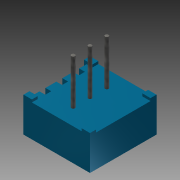
# Autodesk Inventor part: BasePotenciometro
Saved by Autodesk Inventor 2013 (Build 170138000, 138)
## iProperties
Created: 2013-06-26
Part Number: BasePotenciometro
Material: Genérico
Document SubType Name: Modeling
Designer: usuario
Density: 1 g/cm^3
Author: usuario
Autodesk Inventor part; units mm, degrees
ref_plane "YZ Plane" through (0, 0, 0) normal (1, 0, 0) x (0, 1, 0)
ref_plane "XZ Plane" through (0, 0, 0) normal (0, 1, 0) x (-1, 0, 0)
ref_plane "XY Plane" through (0, 0, 0) normal (0, 0, 1) x (1, 0, 0)
sketch "Boceto1" plane through (0, 0, 0) normal (0, 0, 1) x (1, 0, 0)
  line L0 (-4.78, 4.78) -> (4.78, 4.78)
  line L1 (4.78, 4.78) -> (4.78, -4.78)
  line L2 (4.78, -4.78) -> (-4.78, -4.78)
  line L3 (-4.78, -4.78) -> (-4.78, 4.78)
  line L4 (-4.78, 4.78) -> (4.78, -4.78) construction
  line L5 (4.78, 4.78) -> (-4.78, -4.78) construction
  point P0 (0, 0)
  dimension "d0" = 9.56
  dimension "d1" = 9.56
  constraints: 12 end point, 2 midpoint, 2 parallel, 1 horizontal, 1 perpendicular
  measures "d0" distance of L1.end L2.end
  measures "d1" distance of L0.end L1.end
extrude "Extrusión1" add sketch "Boceto1" along normal mid plane 4.6
sketch "Boceto2" plane through (0, 0, 2.3) normal (0, 0, 1) x (1, 0, 0)
  line L0 (-4.78, 4.78) -> (-3.58, 4.78)
  line L1 (-3.58, 4.78) -> (-3.58, 3.92)
  line L2 (-3.58, 3.92) -> (-4.78, 3.92)
  line L3 (-4.78, 3.92) -> (-4.78, 4.78)
  point P0 (0, 0)
  dimension "d4" = 1.2
  dimension "d5" = 0.86
  constraints: 8 end point, 2 parallel, 1 horizontal, 1 perpendicular
  measures "d4" distance of L1.end L2.end
  measures "d5" distance of L0.end L1.end
extrude "Extrusión2" add sketch "Boceto2" along normal blind 0.37
mirror "Simetría1" about plane through (0, 0, 0) normal (0, 1, 0) of "Extrusión2"
mirror "Simetría2" about plane through (0, 0, 0) normal (1, 0, 0) of "Extrusión2", "Simetría1"
sketch "Boceto5" plane through (0, 0, 2.3) normal (0, 0, 1) x (1, 0, 0)
  line L0 (-3.58, 3.92) -> (-4.78, 3.92) projected
  line L1 (-4.78, -3.92) -> (-4.41, -3.92)
  line L2 (-4.41, -3.92) -> (-4.41, 3.92)
  line L3 (-4.41, 3.92) -> (-4.78, 3.92)
  line L4 (-4.78, 3.92) -> (-4.78, -3.92)
  point P0 (0, 0)
  dimension "d21" = 0.37
  constraints: 8 end point, 2 parallel, 1 horizontal, 1 perpendicular, 1 point on line
  measures "d21" distance of L3.end L2.end
extrude "Extrusión4" cut sketch "Boceto5" against normal through all
sketch "Boceto6" plane through (0, 0, 2.3) normal (0, 0, 1) x (1, 0, 0)
  line L0 (-4.41, 3.92) -> (-4.41, -3.92) projected
  line L1 (-4.41, -3.92) -> (-3.58, -3.92) projected
  line L2 (-3.58, -2.85) -> (-3.58, -1.99)
  line L3 (-3.58, -1.99) -> (-4.41, -1.99)
  line L4 (-4.41, -2.85) -> (-3.58, -2.85)
  line L5 (-3.58, -4.78) -> (-4.78, -4.78) projected
  point P0 (0, 0)
  dimension "d24" = 1.93
  dimension "d25" = 0.86
  dimension "d26" = 0.86
  constraints: 6 end point, 2 point on line, 1 parallel, 1 perpendicular
  measures "d24" distance of L5.start L2.start
  measures "d25" distance of L2.start L2.end
  measures "d26" distance between parallel lines of L5 L1
extrude "Extrusión5" cut sketch "Boceto6" against normal through all
mirror "Simetría3" about plane through (0, 0, 0) normal (0, 1, 0) of "Extrusión5"
sketch "Boceto7" plane through (0, 0, 2.3) normal (0, 0, 1) x (1, 0, 0)
  line L0 (-3.58, 1.99) -> (-4.41, 1.99) projected
  line L1 (-4.41, 1.99) -> (-4.41, -1.99) projected
  line L2 (-4.41, -1.99) -> (-3.58, -1.99) projected
  line L3 (-3.58, -2.85) -> (-4.41, -2.85) projected
  line L4 (-3.58, 2.85) -> (-3.58, 1.99) projected
  line L5 (-4.41, -0.43) -> (-3.58, -0.43)
  line L6 (-3.58, -0.43) -> (-3.58, 0.43)
  line L7 (-3.58, 0.43) -> (-4.41, 0.43)
  point P0 (0, 0)
  dimension "d29" = 3.98
  dimension "d30" = 0.86
  dimension "d31" = 0.86
  dimension "d32" = 1.56
  dimension "d33" = 1.56
  constraints: 6 end point, 3 perpendicular, 2 point on line
  measures "d29" distance between parallel lines of L0 L2
  measures "d30" distance between parallel lines of L2 L3
  measures "d31" distance of L5.end L6.end
  measures "d32" distance between parallel lines of L5 L2
  measures "d33" distance between parallel lines of L0 L7
extrude "Extrusión6" cut sketch "Boceto7" against normal through all
sketch "Boceto8" plane through (0, 0, -2.3) normal (0, 0, -1) x (-1, 0, 0)
  circle A0 centre (0, 0) radius 0.5
  dimension "d36" = 1
  constraints: 1 centre point, 1 coincident
  measures "d36" diameter of A0
hole "Hole1" at (0, 0, -2.3) direction (0, 0, 1) diameter 1 depth 2
sketch "Boceto9" plane through (0, 0, 2.3) normal (0, 0, 1) x (1, 0, 0)
  circle A0 centre (0, -2.42) radius 0.25
  circle A1 centre (0, 0) radius 0.25
  circle A2 centre (0, 2.42) radius 0.25
  dimension "d44" = 0.5
  dimension "d45" = 0.5
  dimension "d47" = 0.5
  constraints: 3 centre point, 1 coincident
  measures "d44" diameter of A0
  measures "d45" diameter of A1
  measures "d47" diameter of A2
extrude "Extrusión7" add sketch "Boceto9" along normal blind 6.5
